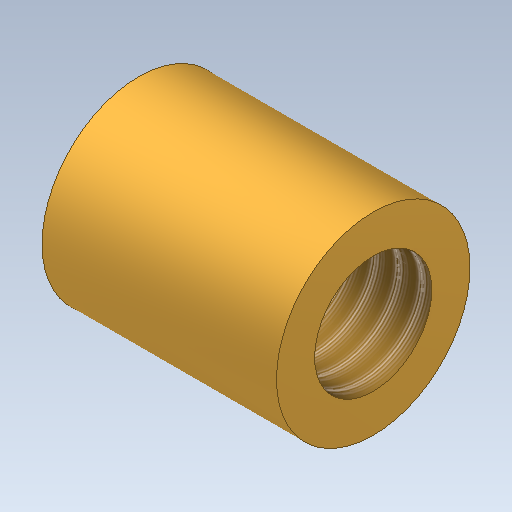
# Autodesk Inventor part: InsertNut_M2_4mm_D3.3
Saved by Autodesk Inventor 2021 (Build 250183000, 183)
## iProperties
Created: 2021-01-29
Part Number: InsertNut_M2_4mm_D3.3
Material: 真鍮、ソフト イエロー
Document SubType Name: Modeling
Designer: yuta2
Density: 8.47 g/cm^3
Appearance: 真鍮 - サテン
Author: yuta2
Autodesk Inventor part; units mm, degrees
ref_plane "YZ Plane" through (0, 0, 0) normal (1, 0, 0) x (0, 1, 0)
ref_plane "XZ Plane" through (0, 0, 0) normal (0, 1, 0) x (-1, 0, 0)
ref_plane "XY Plane" through (0, 0, 0) normal (0, 0, 1) x (1, 0, 0)
sketch "スケッチ1" plane through (0, 0, 0) normal (1, 0, 0) x (0, 1, 0)
  circle A0 centre (0, 0) radius 1
  circle A1 centre (0, 0) radius 1.65
  dimension "d0" = 2
  dimension "d1" = 3.3
  constraints: 2 centre point, 2 coincident
  measures "d0" diameter of A0
  measures "d1" diameter of A1
extrude "押し出し1" add sketch "スケッチ1" along normal blind 4
thread "ねじ1" size "M2x0.4" class "6H" standard "ANSI Metric M Profile" full length
